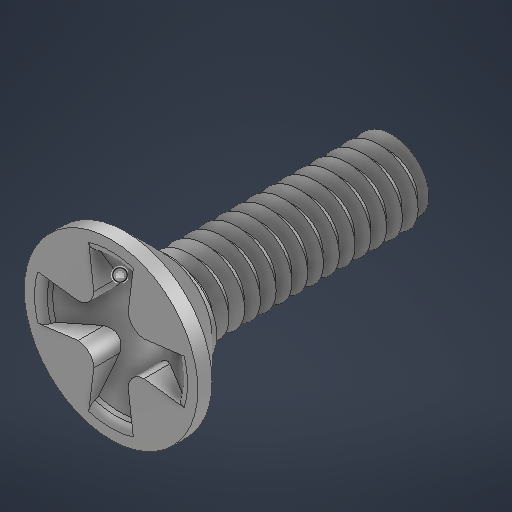
# Autodesk Inventor part: AS 1427 H - Metric M3 x0.5 ALTERADO
Saved by Autodesk Inventor 2025.2 (Build 292293000, 293)
## iProperties
Created: 2024-12-01
Part Number: AS 1427 H - Metric M3 x0.5 ALTERADO
Material: Generic
Document SubType Name: Modeling
Designer: Tiago
Density: 1 g/cm^3
Appearance: Anodized - Light Gray
Author: Tiago
Autodesk Inventor part; units mm, degrees
ref_plane "YZ Plane" through (0, 0, 0) normal (1, 0, 0) x (0, 1, 0)
ref_plane "XZ Plane" through (0, 0, 0) normal (0, 1, 0) x (-1, 0, 0)
sketch "Sketch2" plane through (0, 0, 0) normal (0, 1, 0) x (-1, 0, 0)
  line L0 (0, -1.5) -> (0, -10)
  line L1 (0, -10) -> (-1.5, -8.6)
  line L2 (-1.5, -8.6) -> (-1.5, -1.7)
  line L3 (-1.5, -1.7) -> (-2.75, -0.45)
  line L4 (-2.75, -0.45) -> (-2.75, 0)
  line L5 (-2.75, 0) -> (-2.25, 0)
  line L6 (-2.1218, -0.275) -> (0, -1.5)
  line L7 (-2.25, 0) -> (-2.1218, -0.275)
  line L8 (0, -10) -> (0, -9)
  line L9 (0, -9) -> (-1.0714, -9)
  point P0 (0, 0)
  point P1 (-2.5, 0)
  dimension "d0" = 3
  dimension "dk" = 5.5
  dimension "d3" = 4.5
  dimension "d4" = 60
  dimension "d5" = 25
  dimension "d6" = 1.5
  dimension "k" = 1.7
  dimension "d8" = 45
  dimension "L" = 10
  dimension "d10" = 1.4
  dimension "d53" = 1
  constraints: 20 end point, 4 point on line, 2 parallel, 1 horizontal, 1 midpoint, 1 perpendicular, 1 vertical
  measures "d0" diameter of L2 L0
  measures "dk" diameter of L4 L0
  measures "d3" diameter of L5.end L0
  measures "d4" angle of L6 L0
  measures "d5" angle of L0 L7
  measures "d6" vertical distance of L0.start point (-2.5, 0)
  measures "k" vertical distance of L2.end L4.end
  measures "d8" angle of L0 L3
  measures "L" distance from line of L0.end L5
  measures "d10" vertical distance of L0.end L1.end
  measures "d53" distance of L0.end L8.end
revolve "Revolution1" add sketch "Sketch2" angle 360 about axis through (0, 0, -1.5) along (0, 0, -1) contours L0 L9 L1 L2 L3 L4 L5 L7 L6
sketch "Sketch3" plane through (0, 0, 0) normal (0, 0, 1) x (1, 0, 0)
  line L0 (0, 3.85) -> (0, -3.85) projected
  line L1 (-4.0894, 0) -> (5.2866, 0) projected
  circle A0 centre (0, 0) radius 2.25 projected
  line L2 (0, 2.25) -> (0.6965, 2.25) construction
  line L3 (0, 2.25) -> (-0.697, 2.25)
  line L4 (2.25, 0) -> (2.25, 0.6965) construction
  line L5 (2.25, 0) -> (2.25, -0.6965) construction
  line L6 (-0.697, 2.25) -> (-0.697, 2.1393)
  line L7 (0.6965, 2.25) -> (0.6965, 2.1395)
  line L8 (2.1395, 0.6965) -> (2.25, 0.6965)
  arc A1 (2.25, 0.6965) -> (0.6965, 2.25) centre (0, 0) ccw
  line L9 (-0.697, -0.0785) -> (-0.697, 0.2705) construction
  line L10 (-0.5455, 1.0455) -> (0.5455, 1.0455) construction
  line L11 (-0.697, 2.25) -> (-0.5455, 1.0455)
  line L12 (0.6965, 2.25) -> (0.5455, 1.0455)
  line L13 (0.6965, 0.6965) -> (1.0455, 0.6965) construction
  line L14 (1.0455, -0.5455) -> (1.0455, 0.5455) construction
  line L15 (1.0455, 0.5455) -> (2.25, 0.6965)
  line L16 (1.0455, -0.5455) -> (2.25, -0.6965)
  line L17 (0.6965, 0.6965) -> (0.6965, 1.0455) construction
  arc A2 (0.5455, 1.0455) -> (1.0455, 0.5455) centre (1.0617, 1.0617) ccw
  line L18 (-2.25, 0) -> (-2.25, 0.6965) construction
  arc A3 (-0.6965, 2.25) -> (-2.25, 0.6965) centre (0, 0) ccw
  line L19 (-1.0455, 0.5455) -> (-2.25, 0.6965)
  arc A4 (-1.0455, 0.5455) -> (-0.5455, 1.0455) centre (-1.0617, 1.0617) ccw
  line L20 (0, -2.25) -> (0.6965, -2.25) construction
  line L21 (0, -2.25) -> (-0.697, -2.25) construction
  line L22 (-0.697, -2.25) -> (-0.5455, -1.0455)
  line L23 (0.6965, -2.25) -> (0.5455, -1.0455)
  arc A5 (1.0455, -0.5455) -> (0.5455, -1.0455) centre (1.0617, -1.0617) ccw
  arc A6 (-0.5455, -1.0455) -> (-1.0455, -0.5455) centre (-1.0617, -1.0617) ccw
  line L24 (-2.25, 0) -> (-2.25, -0.6965) construction
  line L25 (-1.0455, -0.5455) -> (-2.25, -0.6965)
  arc A7 (-2.25, -0.6965) -> (-0.697, -2.25) centre (0.5801, 0.5797) ccw
  arc A8 (0.6965, -2.25) -> (3.6055, -0.117) centre (0.6574, 0.8535) ccw
  point P0 (0, 0)
  point P1 (0, 1.0455)
  point P2 (1.0455, 0)
  point P3 (-2.1438, -0.6832)
  point P4 (-0.6836, -2.1436)
  point P5 (-0.6836, 2.1436)
  point P6 (-2.1438, 0.6832)
  point P7 (0.6832, -2.1438)
  point P8 (2.1438, -0.6832)
  point P9 (2.1438, 0.6832)
  point P10 (0.6832, 2.1438)
  dimension "d12" = 0.6965
  dimension "d13" = 0.697
  dimension "d14" = 0.6965
  dimension "d15" = 0.6965
  dimension "d17" = 0.349
  dimension "d20" = 1.091
  dimension "d21" = 0.349
  dimension "d22" = 1.091
  constraints: 48 end point, 23 point on circle, 14 symmetric about line, 8 centre point, 6 point on line, 4 horizontal, 4 vertical, 2 midpoint, 2 perpendicular, 2 tangent, 4 other
  measures "d12" distance of L2.start L2.end
  measures "d13" distance of L2.start L3.end
  measures "d14" distance of L4.start L4.end
  measures "d15" distance of L4.start L5.end
  measures "d17" distance of L9.start L9.end
  measures "d20" distance of L10.start L10.end
  measures "d21" distance of L13.start L13.end
  measures "d22" distance of L14.start L14.end
extrude "Extrusion1" add sketch "Sketch3" against normal up to next contours A0 L15 A2 L12 | L11 A4 L19 A0 | A0 L25 A6 L22 | L23 A5 L16 A0
fillet "Fillet1" radius 0.274 4 edges at (-0.0002, 2.25, 0) (2.25, 0, 0) (-0.0002, -2.25, 0) (-2.25, 0, 0)
sketch "Sketch4" plane through (0, 0, 0) normal (0, 1, 0) x (-1, 0, 0)
  line L0 (0, -12.0072) -> (0, 2.0434) projected
  line L1 (-2.75, -0.45) -> (-1.5, -1.7) projected
  line L2 (2.75, -0.45) -> (1.5, -1.7) projected
  line L3 (1.5, -1.7) -> (1.5, -8.6) projected
  line L4 (1.5, -8.6) -> (1.0714, -9) projected
  line L5 (-1.0714, -9) -> (-1.5, -8.6) projected
  line L6 (-1.5, -8.6) -> (-1.5, -1.7) projected
  line L7 (-1.5, -1.7) -> (-2.75, -0.45) projected
  line L8 (-2.75, -0.45) -> (-2.75, 0) projected
  line L9 (-2.75, 0) -> (-2.4246, 0) projected
  arc A0 (-2.1762, -0.1582) -> (-2.4246, 0) centre (-2.4246, -0.274) ccw projected
  line L10 (-2.1762, -0.1582) -> (-2.1218, -0.275) projected
  line L11 (-2.1218, -0.275) -> (0, -1.5) projected
  line L12 (0, -1.5) -> (2.1218, -0.275) projected
  line L13 (2.1218, -0.275) -> (2.1762, -0.1582) projected
  arc A1 (2.4246, 0) -> (2.1762, -0.1582) centre (2.4246, -0.274) ccw projected
  line L14 (2.4246, 0) -> (2.75, 0) projected
  line L15 (2.75, 0) -> (2.75, -0.45) projected
  line L16 (-1.5, -8.85) -> (-1.5, -9.6834)
  line L17 (-1.5, -9.6834) -> (-0.8865, -9.3292)
  line L18 (-0.8865, -9.3292) -> (-0.8865, -9.2042)
  line L19 (-1.5, -8.85) -> (-0.8865, -9.2042)
  line L20 (-1.5, -9.2667) -> (-0.8865, -9.2667)
  line L21 (0, -10) -> (0, -9)
  line L22 (2.1429, -9) -> (-2.1429, -9)
  line L23 (1.0714, -9) -> (-1.0714, -9) projected
  point P0 (0, 0)
  point P1 (-1.1933, -9.2667)
  dimension "d26" = 60
  dimension "d" = 1.773
  dimension "d28" = 0.25
  dimension "d29" = 0.125
  constraints: 14 end point, 4 midpoint, 2 horizontal, 2 point on line, 1 equal length, 1 parallel, 1 vertical, 1 other
  measures "d26" angle of L19 L17
  measures "d" diameter of L18 L0
  measures "d28" distance of L5.end L16.start
  measures "d29" distance of L17.end L18.end
coil "Coil1" sketch "Sketch4" operation cut axis through (0, 0, -10) along (0, 0, 1) pitch 0.5 turns 14.4 hand right contours L20 L18 L17 L16 | L16 L22 L19 L18 L20 | L16 L19 L22
ref_plane "Work Plane1" through (0, 0, -3) normal (0, 0, 1) x (1, 0, 0)
body "Solid1"
